# Autodesk Inventor part: BS 3692 - M30 x 90
Saved by Autodesk Inventor 2020.1 (Build 241239000, 239)
## iProperties
Comments: To add or edit properties for Autodesk Inventor files, use iProperties.
Shininess: 64.0
Length Units: 11269
Angle Units: 11279
Time Units: 11290
Mass Units: 11283
Length Display Precision: 3
Angle Display Precision: 2
Compacted: True
Alert: To add or edit properties for Autodesk Inventor files, use iProperties.
Created: 2003-05-03
Part Number: BS 3692 - M30 x 90
Vendor: Autodesk Inc.
Document SubType Name: Modeling
Designer: Stephen Hooper
Material: Generic
Description: Hex-Head Bolt
Standard: BS 3692
Manufacturer: Standard
Standards Organization: Custom
Density: 1 g/cm^3
Appearance: Default
Density: 0.0
Volumn: 0.0
Area: 0.0
PropertySet Name: Model Information
Control State: 0
Master: False
Checked Out: False
EGR: 1
Author: Stephen Hooper
Revision Number: 5
Autodesk Inventor part; units mm, degrees
ref_plane "YZ Plane" through (0, 0, 0) normal (1, 0, 0) x (0, 1, 0)
ref_plane "XZ Plane" through (0, 0, 0) normal (0, 1, 0) x (-1, 0, 0)
ref_plane "XY Plane" through (0, 0, 0) normal (0, 0, 1) x (1, 0, 0)
sketch "Sketch1" plane through (0, 0, 0) normal (0, 0, 1) x (1, 0, 0)
  line L0 (0, 20.7) -> (0, 15)
  line L1 (29, 15) -> (95, 15)
  line L2 (95, 15) -> (95, 0)
  line L3 (95, 0) -> (-0.5001, 0)
  line L4 (-10.0501, 0) -> (123.65, 0) projected
  line L5 (-0.5001, 0) -> (-0.5001, 20.7)
  line L6 (-0.5001, 20.7) -> (0, 20.7)
  line L7 (29, 15) -> (26.8528, 15)
  line L8 (26.8528, 15) -> (0, 15)
  line L9 (0, -2.07) -> (0, 26.91) projected
  dimension "d0" = 95
  dimension "d1" = 66
  dimension "d2" = 30
  dimension "d9" = 0.5001
  dimension "d10" = 41.4
  dimension "d13" = 2.1472
  dimension "d14" = 30
  constraints: 16 end point, 2 collinear, 2 perpendicular, 1 parallel
  measures "d0" distance between parallel lines of L2 L0
  measures "d1" distance from line of L1.start L2
  measures "d2" diameter of L1 L3
  measures "d9" distance between parallel lines of L5 L0
  measures "d10" diameter of L6 L3
  measures "d13" distance of L1.start L7.end
  measures "d14" diameter of L8 L3
revolve "Body" add sketch "Sketch1" angle 360 about axis through (95, 0, 0) along (-1, 0, 0)
sketch "Sketch2" plane through (-0.5001, 0, 0) normal (-1, 0, 0) x (0, 0, 1)
  line L0 (0, 26.5581) -> (23, 13.2791)
  line L1 (23, 13.2791) -> (23, -13.2791)
  line L2 (23, -13.2791) -> (0, -26.5581)
  line L3 (0, -26.5581) -> (-23, -13.2791)
  line L4 (-23, -13.2791) -> (-23, 13.2791)
  line L5 (-23, 13.2791) -> (0, 26.5581)
  point P0 (0, 0)
  point P1 (0, 0)
  dimension "d11" = 46
  constraints: 12 end point, 1 coincident, 1 vertical, 11 other
  measures "d11" distance between parallel lines of L4 L1
extrude "Head" add sketch "Sketch2" along normal blind 18.76
sketch "Sketch4" plane through (0, 0, 0) normal (0, 0, 1) x (1, 0, 0)
  line L0 (-19.2601, 23) -> (-19.2601, 26.5581)
  line L1 (-19.2601, 26.5581) -> (-17.2058, 26.5581)
  line L2 (-17.2058, 26.5581) -> (-19.2601, 23)
  line L3 (-21.1361, 0) -> (5.1279, 0) projected
  line L4 (-0.5001, 26.5581) -> (-19.2601, 26.5581) projected
  line L5 (-19.2601, 13.2791) -> (-19.2601, 26.5581) projected
  dimension "d5" = 30
  dimension "d19" = 46
  constraints: 6 end point, 2 collinear, 1 perpendicular, 1 vertical
  measures "d5" angle of L2 L0
  measures "d19" diameter of L0.start L3
revolve "Chamfer1" cut sketch "Sketch4" angle 360 about axis through (-10, 0, 0) along (1, 0, 0)
thread "Thread" size "M30x3.5" class "6g" standard "ISO Metric profile" length 66
chamfer "Chamfer2" distance 2.1471 distance2 2.1472 1 edges at (95, -15, 0) measured on face at (95, -3.9999, 1.1966)
equation "\"d0\" = NLG"
equation "\"d1\" = GEL"
equation "\"d2\" = GD"
equation "\"d10\" = SD2"
equation "\"d14\" = BDM"
equation "\"d11\" = SW"
equation "\"d3\" = KOH - SD"
equation "\"d5\" = ANG1"
equation "\"d19\" = SW0"
equation "\"d15\" = GEL"
equation "\"d6\" = -0.5 * SPD + 0.5 * GD"
equation "\"NLG\" = 95"
equation "\"GD\" = NND"
equation "\"BDM\" = NND"
equation "\"KOH\" = 19.26"
equation "\"GEL\" = 66"
equation "\"SW\" = 46"
equation "\"SW0\" = 46"
equation "\"SPD\" = NND - 1.2269 * TPU"
equation "\"SD2\" = 0.9 * SW"
equation "\"SD\" = 0.5"
equation "\"ANG1\" = 30deg"
equation "\"GAL\" = 0.61345 * TPU"
equation "\"GUL\" = 0.61345 * TPU"
equation "\"RR\" = 1.7"
equation "\"d20\" = -NLG"
equation "\"TOA\" = 30deg"
equation "\"PTC\" = TPU"
equation "\"GD1\" = THREADDIA - 1.2269 * TPU"
equation "\"TPU\" = 3.5"
equation "\"E0\" = 1.155 * SW"
equation "\"SDH\" = 44.98"
equation "\"NND\" = 30"
equation "\"THREADDIA\" = 30"
body "Solid1"
